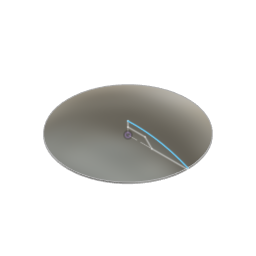
MPB2015 Feet v4 (Autodesk Fusion 360 design; units mm, degrees)
Autodesk Fusion 360 part; units mm, degrees
sketch "2015 Profile" plane through (0, 0, 0) normal (0, 1, 0) x (1, 0, 0) in component "Macbook Pro Pad"
  line L0 (0, -1) -> (0, -1.75)
  line L1 (0, -1) -> (2.5, -1)
  line L2 (3.5, 0) -> (8.75, 0)
  line L3 (0, 0) -> (3.5, 0) construction
  line L4 (0, 0) -> (0, -1) construction
  line L5 (8.75, 0) -> (8.75, -0.2)
  arc A0 (0, -1.75) -> (8.75, -0.2) centre (0.9618, 18.2928) ccw
  line L6 (3.5, 0) -> (2.5, -1)
  dimension "d1" = 1.75
  dimension "d2" = 8.75
  dimension "d3" = 3.5
  dimension "d6" = 0.2
  dimension "d7" = 2.5
  dimension "d8" = 1
  constraint coincident L3.start L4.start
  constraint vertical L0
  constraint perpendicular L0 L1
  constraint horizontal L2
  constraint horizontal L3
  constraint vertical L4
  constraint perpendicular L2 L5
  measures "d1" distance of L3.start L0.end
  measures "d2" distance of L3.start L2.end
  measures "d3" distance of L3.start L2.start
  measures "d6" distance of L2.end L5.end
  measures "d7" distance of L0.start L1.end
  measures "d8" distance of L3.start L0.start
revolve "Revolve2" add sketch "2015 Profile" angle 360 about axis through (0, 0, 1) along (0, 0, 1) in component "Macbook Pro Pad"
component "Macbook Pro Pad" placed x (1, 0, 0) y (0, 1, 0) z (0, 0, 1) at (0, 0, 0)
equation "d2 = ( 17.5 / 2 ) * 1 mm"
equation "d3 = ( 7 / 2 ) * 1 mm"
named bodies: "2015Feet"
